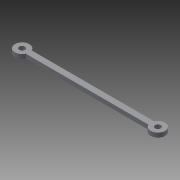
# Autodesk Inventor part: Restrain_Pin_1
Saved by Autodesk Inventor 2015 (Build 190159000, 159)
## iProperties
Created: 2016-07-06
Part Number: Restrain_Pin_1
Material: Generic
Document SubType Name: Modeling
Designer: Neelotpal Nag
Density: 1 g/cm^3
Appearance: Default
Author: Neelotpal Nag
Autodesk Inventor part; units mm, degrees
ref_plane "YZ Plane" through (0, 0, 0) normal (1, 0, 0) x (0, 1, 0)
ref_plane "XZ Plane" through (0, 0, 0) normal (0, 1, 0) x (-1, 0, 0)
ref_plane "XY Plane" through (0, 0, 0) normal (0, 0, 1) x (1, 0, 0)
sketch "Sketch1" plane through (0, 0, 0) normal (0, 0, 1) x (1, 0, 0)
  circle A0 centre (0, 0) radius 1
  circle A1 centre (47.0377, -0.0423) radius 1
  arc A2 (2.2923, 0.9976) -> (2.2904, -1.0021) centre (0, 0) ccw
  arc A3 (44.7455, -1.0402) -> (44.7473, 0.9598) centre (47.0377, -0.0423) ccw
  line L0 (0, -2) -> (0, 1)
  line L1 (48.4179, 2.0423) -> (48.671, 2.0423)
  line L2 (48.671, -1.9577) -> (48.6442, -1.9577)
  line L3 (48.671, 2.0423) -> (48.671, 1.8505)
  line L4 (48.671, -1.935) -> (48.671, -1.9577)
  line L5 (0, 1) -> (0.0018, 1)
  line L6 (2.2923, 0.9976) -> (44.7473, 0.9598)
  line L7 (47.0404, -1.0422) -> (47.0368, -1.0423)
  line L8 (44.7455, -1.0402) -> (2.2904, -1.0021)
  dimension "d0" = 2
  dimension "d1" = 2
  dimension "d2" = 5
  dimension "d3" = 5
  dimension "d5" = 4
  constraints: 18 end point, 12 point on circle, 5 coincident, 5 perpendicular, 4 centre point, 2 tangent, 1 horizontal
  measures "d0" diameter of A0
  measures "d1" diameter of A1
  measures "d2" diameter of A2
  measures "d3" diameter of A3
  measures "d5" distance of L1.end L2.start
extrude "Extrusion1" add sketch "Sketch1" along normal blind 1.5 contours L6 A3 L8 A2
body "Solid1"
